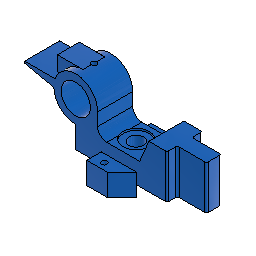
Design 13 v1 (Autodesk Fusion 360 design; units mm, degrees)
Autodesk Fusion 360 part; units mm, degrees
sketch "Sketch1" plane through (0, 0, 0) normal (0, 0, 1) x (1, 0, 0)
  line L0 (50, -24) -> (-50, -24)
  line L1 (-50, -24) -> (-50, 24)
  line L2 (-50, 24) -> (50, 24)
  line L3 (50, 24) -> (50, -24)
  line L4 (50, -24) -> (-50, 24) construction
  line L5 (-50, -24) -> (50, 24) construction
  dimension "d1" = 100
  dimension "d2" = 48
  constraint horizontal L0
  constraint perpendicular L0 L1
  constraint parallel L0 L2
  constraint parallel L1 L3
  constraint coincident L4 origin
  constraint coincident L5 origin
  measures "d1" distance of L1.end L2.end
  measures "d2" distance of L0.end L1.end
extrude "Extrude1" add sketch "Sketch1" along normal blind 30
sketch "Sketch2" plane through (0, -24, 0) normal (0, -1, 0) x (1, 0, 0)
  line L0 (-50, 0) -> (50, 0)
  line L1 (50, 0) -> (50, 30)
  line L2 (50, 30) -> (-50, 30)
  line L3 (-50, 30) -> (-50, 0)
  line L4 (50, 0) -> (75, 0)
  line L5 (75, 0) -> (75, 60)
  line L6 (75, 60) -> (50, 60)
  line L7 (50, 60) -> (50, 0)
  line L8 (75, 60) -> (115, 60)
  line L9 (115, 60) -> (115, 0)
  line L10 (115, 0) -> (75, 0)
  line L11 (75, 0) -> (75, 60)
  line L12 (50, 60) -> (37.5, 30)
  circle A0 centre (-50, 60) radius 30
  circle A1 centre (-50, 60) radius 20
  line L13 (-15, 0) -> (33, 0)
  line L14 (33, 0) -> (33, 15)
  line L15 (33, 15) -> (-15, 15)
  line L16 (-15, 15) -> (-15, 0)
  line L17 (-50, 60) -> (-50, 70)
  line L18 (-50, 70) -> (-120, 70)
  line L19 (-120, 70) -> (-120, 67.5)
  line L20 (-120, 67.5) -> (-50, 52.5)
  line L21 (-50, 52.5) -> (-50, 60)
  line L22 (-50, 90) -> (-85, 90)
  line L23 (-85, 90) -> (-85, 70)
  line L24 (-85, 70) -> (-50, 70)
  line L25 (-50, 70) -> (-50, 90)
  line L26 (-20, 60) -> (-20, 30)
  dimension "d5" = 25
  dimension "d6" = 60
  dimension "d7" = 40
  dimension "d8" = 60
  dimension "d9" = 40
  dimension "d10" = 48
  dimension "d11" = 15
  dimension "d12" = 10
  dimension "d13" = 70
  dimension "d14" = 7.5
  dimension "d15" = 35
  dimension "d16" = 12.5
  constraint horizontal L4
  constraint vertical L5
  constraint horizontal L6
  constraint vertical L7
  constraint coincident L0.end L1.start
  constraint horizontal L8
  constraint vertical L9
  constraint horizontal L10
  constraint vertical L11
  constraint coincident L2 L12.end
  constraint coincident L2.end A0
  constraint concentric A0 A1
  constraint horizontal L13
  constraint vertical L14
  constraint horizontal L15
  constraint vertical L16
  constraint coincident L0 L13.start
  constraint coincident A0.centre A1.centre
  constraint vertical L17
  constraint perpendicular L17 L18
  constraint perpendicular L18 L19
  constraint parallel L17 L21
  constraint horizontal L22
  constraint vertical L23
  constraint horizontal L24
  constraint vertical L25
  constraint midpoint L18 L23.end
  constraint coincident A0 L22.start
  constraint coincident A0 L26.start
  constraint coincident L2 L26.end
  constraint tangent A0 L26
  constraint perpendicular L2 L26
  measures "d5" distance of L0.end L4.end
  measures "d6" distance of L0.end L6.end
  measures "d7" distance of L5.end L8.end
  measures "d8" diameter of A0
  measures "d9" diameter of A1
  measures "d10" distance of L13.start L13.end
  measures "d11" distance of L13.start L15.end
  measures "d12" distance of A0.centre L17.end
  measures "d13" distance of L17.end L18.end
  measures "d14" distance of L20.end A0.centre
  measures "d15" distance of L0.start L13.start
  measures "d16" distance of L1.end L12.end
extrude "Extrude2" add sketch "Sketch2" against normal blind 48 contours L2 A0 L26 | A0 A1 L20 L25 | A0 L18 L19 L20 L24 | A0 A1 L18 L20 L24 | L1 L4 L5 L6 L7 L11 | L2 L7 L12 | A0 A1 L18 L24 L25
extrude "Extrude3" add sketch "Sketch2" against normal blind 20 from surface at -14 contours L5 L8 L9 L10 L11
extrude "Extrude4" add sketch "Sketch2" against normal blind 30 from surface at -10 contours A0 L18 L22 L23 L24
extrude "Extrude5" add sketch "Sketch2" along normal blind 20 contours L0 L13 L14 L15 L16
sketch "Sketch3" plane through (0, 0, 15) normal (0, 0, 1) x (-1, 0, 0)
  line L0 (-33, 24) -> (15, 24)
  line L1 (15, 24) -> (15, 44)
  line L2 (15, 44) -> (-33, 44)
  line L3 (-33, 44) -> (-33, 24)
  line L4 (-33, 24) -> (-3.4619, 53.5381)
  line L5 (-33, 24) -> (8.7732, 24) construction
  circle A0 centre (0, 35) radius 3.75
  dimension "d27" = 45
  dimension "d28" = 7.5
  dimension "d29" = 15
  constraint horizontal L5
  constraint coincident L0.start L3.end
  measures "d27" angle of L4 L5
  measures "d28" diameter of A0
  measures "d29" distance of L1 A0.centre
extrude "Extrude6" cut sketch "Sketch3" against normal blind 40 contours L2 L3 L4 | A0
mirror "Mirror1" about plane through (0, 0, 0) normal (0, 0, -1) of "Extrude5", "Extrude6"
mirror "Mirror2" about plane through (0, 0, 0) normal (0, 1, 0) of "Extrude5", "Mirror1"
hole "Hole1" at (-50, 1, 90) direction (0, 0, -1) diameter 7.5 depth 30 tip angle 180
hole "Hole2" at (8.75, 0, 30) direction (0, 0, -1) diameter 20 depth 60 tip angle 180 counterbore diameter 36 counterbore depth 2.5
fillet "Fillet1" radius 12.5 1 edges at (-20, 0, 30)
fillet "Fillet2" radius 2.5 6 edges at (75, -10, 30) (75, 10, 30) (75, 24, 30) (115, 10, 30) (115, -10, 30) (75, -24, 30)
